Autodesk Inventor part; units mm, degrees
note: some values were not read from the file. Chosen so that the rebuilt part matches the saved one: direction of "Hole2".
(part 6 of 20)
  line L798 (-10086.965544, -10011.716706) -> (-10086.965599, -10011.716869)
  line L799 (-10086.460356, -10011.664008) -> (-10086.460302, -10011.663845)
  line L800 (-10067.443775, -10022.078908) -> (-10063.849959, -10021.096991)
  line L801 (-10063.849959, -10017.096991) -> (-10067.443775, -10016.115074)
  line L802 (-10063.849959, -10021.096991) -> (-10063.849959, -10017.096991)
  line L803 (-10064.171558, -10021.472431) -> (-10062.806719, -10021.096991)
  line L804 (-10062.806719, -10017.096991) -> (-10064.162196, -10016.724126)
  line L805 (-10062.806719, -10021.096991) -> (-10062.806719, -10017.096991)
  line L806 (-10064.538813, -10027.464433) -> (-10072.041452, -10028.601455)
  line L807 (-10064.538833, -10027.464382) -> (-10064.538813, -10027.464433)
  line L808 (-10072.041471, -10028.601404) -> (-10064.538833, -10027.464382)
  line L809 (-10072.041452, -10028.601455) -> (-10072.041471, -10028.601404)
  line L810 (-10064.074644, -10023.491407) -> (-10066.019072, -10022.707953)
  line L811 (-10064.074624, -10023.491459) -> (-10064.074644, -10023.491407)
  line L812 (-10077.559629, -10027.956681) -> (-10072.041471, -10028.601404)
  line L813 (-10077.559609, -10027.956732) -> (-10072.041452, -10028.601455)
  line L814 (-10064.538813, -10027.464433) -> (-10064.074624, -10023.491459)
  line L815 (-10064.538833, -10027.464382) -> (-10064.074644, -10023.491407)
  ellipse E634 centre (-10077.559589, -10027.956784) end of major axis (-10077.055021, -10028.015736) minor radius 0.000049 (-10077.55961, -10027.956732) -> (-10077.792591, -10027.929517) ccw
  ellipse E635 centre (-10077.559589, -10027.956784) end of major axis (-10076.550453, -10028.074688) minor radius 0.000097 (-10077.559631, -10027.956681) -> (-10078.025593, -10027.90225) ccw
  ellipse E636 centre (-10084.064431, -10027.197109) end of major axis (-10085.073566, -10027.079205) minor radius 0.000097 (-10084.530433, -10027.142576) -> (-10085.073566, -10027.079205) ccw
  ellipse E637 centre (-10084.064431, -10027.197109) end of major axis (-10084.568999, -10027.138157) minor radius 0.000049 (-10084.297432, -10027.169842) -> (-10084.568999, -10027.138157) ccw
  line L816 (-10085.073566, -10027.079205) -> (-10085.026899, -10026.679784)
  line L817 (-10077.79259, -10027.929517) -> (-10084.297432, -10027.169842)
  line L818 (-10078.025591, -10027.90225) -> (-10084.530433, -10027.142576)
  line L819 (-10085.073527, -10027.079306) -> (-10085.189452, -10028.072869)
  line L820 (-10084.684884, -10028.131821) -> (-10085.189452, -10028.072869)
  line L821 (-10084.684884, -10028.131821) -> (-10084.56896, -10027.138258)
  line L822 (-10085.073527, -10027.079306) -> (-10084.56896, -10027.138258)
  line L823 (-10085.189452, -10028.072869) -> (-10085.189425, -10028.072939)
  line L824 (-10084.56896, -10027.138258) -> (-10084.568999, -10027.138157)
  line L825 (-10085.073566, -10027.079205) -> (-10085.073527, -10027.079306)
  line L826 (-10065.745685, -10021.096991) -> (-10073.016339, -10023.096991)
  line L827 (-10065.804571, -10021.096991) -> (-10065.745685, -10021.096991)
  line L828 (-10073.075225, -10023.096991) -> (-10065.804571, -10021.096991)
  line L829 (-10073.016339, -10023.096991) -> (-10073.075225, -10023.096991)
  line L830 (-10073.016339, -10015.096991) -> (-10065.745685, -10017.096991)
  line L831 (-10073.075225, -10015.096991) -> (-10073.016339, -10015.096991)
  line L832 (-10065.804571, -10017.096991) -> (-10073.075225, -10015.096991)
  line L833 (-10065.745685, -10017.096991) -> (-10065.804571, -10017.096991)
  line L834 (-10078.593466, -10023.096991) -> (-10073.075225, -10023.096991)
  line L835 (-10078.593466, -10015.096991) -> (-10073.075225, -10015.096991)
  line L836 (-10065.745685, -10021.096991) -> (-10065.745685, -10017.096991)
  line L837 (-10065.804571, -10021.096991) -> (-10065.804571, -10017.096991)
  line L838 (-10078.593466, -10023.096991) -> (-10079.046133, -10023.096991)
  line L839 (-10078.593466, -10015.096991) -> (-10079.046133, -10015.096991)
  line L840 (-10079.046133, -10023.096991) -> (-10079.694033, -10023.096991)
  line L841 (-10079.694033, -10015.096991) -> (-10079.046133, -10015.096991)
  line L842 (-10085.400929, -10014.884409) -> (-10085.478798, -10015.096991)
  line L843 (-10084.974223, -10015.096991) -> (-10084.918326, -10014.944393)
  line L844 (-10085.478798, -10023.096991) -> (-10085.400929, -10023.309573)
  line L845 (-10084.918326, -10023.249589) -> (-10084.974223, -10023.096991)
  line L846 (-10064.074644, -10014.702574) -> (-10064.074624, -10014.702523)
  line L847 (-10066.019072, -10015.486029) -> (-10064.074644, -10014.702574)
  line L848 (-10072.041452, -10009.592527) -> (-10064.538813, -10010.729548)
  line L849 (-10072.041471, -10009.592578) -> (-10072.041452, -10009.592527)
  line L850 (-10064.538833, -10010.7296) -> (-10072.041471, -10009.592578)
  line L851 (-10064.538813, -10010.729548) -> (-10064.538833, -10010.7296)
  line L852 (-10072.041452, -10009.592527) -> (-10077.559609, -10010.237249)
  line L853 (-10077.559629, -10010.237301) -> (-10072.041471, -10009.592578)
  line L854 (-10064.074624, -10014.702523) -> (-10064.538813, -10010.729548)
  line L855 (-10064.074644, -10014.702574) -> (-10064.538833, -10010.7296)
  ellipse E638 centre (-10077.559589, -10010.237198) end of major axis (-10078.064157, -10010.29615) minor radius 0.000049 (-10077.79259, -10010.264465) -> (-10077.559609, -10010.237249) ccw
  ellipse E639 centre (-10077.559589, -10010.237198) end of major axis (-10076.550453, -10010.119294) minor radius 0.000097 (-10078.025593, -10010.291731) -> (-10077.559631, -10010.237301) ccw
  ellipse E640 centre (-10084.064431, -10010.996873) end of major axis (-10085.073566, -10011.114777) minor radius 0.000097 (-10085.073566, -10011.114777) -> (-10084.530433, -10011.051406) ccw
  ellipse E641 centre (-10084.064431, -10010.996873) end of major axis (-10084.568999, -10011.055825) minor radius 0.000049 (-10084.568999, -10011.055825) -> (-10084.297432, -10011.024139) ccw
  line L856 (-10085.026899, -10011.514198) -> (-10085.073566, -10011.114777)
  line L857 (-10077.79259, -10010.264465) -> (-10084.297432, -10011.024139)
  line L858 (-10084.530433, -10011.051406) -> (-10078.025591, -10010.291731)
  line L859 (-10085.189452, -10010.121112) -> (-10085.073527, -10011.114675)
  line L860 (-10084.56896, -10011.055724) -> (-10085.073527, -10011.114675)
  line L861 (-10084.56896, -10011.055724) -> (-10084.684884, -10010.06216)
  line L862 (-10084.684884, -10010.06216) -> (-10085.189452, -10010.121112)
  line L863 (-10085.189425, -10010.121042) -> (-10085.189452, -10010.121112)
  line L864 (-10085.073527, -10011.114675) -> (-10085.073566, -10011.114777)
  line L865 (-10084.568999, -10011.055825) -> (-10084.56896, -10011.055724)
  line L866 (-10081.349998, -10026.695676) -> (-10079.440529, -10026.876667)
  line L867 (-10081.349996, -10026.695712) -> (-10080.62193, -10026.764723)
  ellipse E642 centre (-10081.349994, -10026.695749) end of major axis (-10080.84426, -10026.743685) minor radius 0.000036 (-10081.349998, -10026.695712) -> (-10081.583519, -10026.673581) ccw
  ellipse E643 centre (-10081.349994, -10026.695749) end of major axis (-10080.338527, -10026.791622) minor radius 0.000072 (-10081.350003, -10026.695675) -> (-10081.817045, -10026.651414) ccw
  ellipse E644 centre (-10087.869978, -10026.077987) end of major axis (-10088.881445, -10025.982114) minor radius 0.000072 (-10088.337025, -10026.033654) -> (-10088.881445, -10025.982114) ccw
  ellipse E645 centre (-10087.869978, -10026.077987) end of major axis (-10088.375711, -10026.030051) minor radius 0.000036 (-10088.103502, -10026.05582) -> (-10088.375711, -10026.030051) ccw
  line L868 (-10088.881445, -10025.982114) -> (-10088.665315, -10023.701932)
  line L869 (-10081.583517, -10026.673582) -> (-10088.103502, -10026.05582)
  line L870 (-10081.817041, -10026.651415) -> (-10088.337025, -10026.033654)
  line L871 (-10088.88144, -10025.982186) -> (-10088.975789, -10026.97795)
  line L872 (-10088.470056, -10027.025887) -> (-10088.975789, -10026.97795)
  line L873 (-10088.470056, -10027.025887) -> (-10088.375707, -10026.030122)
  line L874 (-10088.88144, -10025.982186) -> (-10088.375707, -10026.030122)
  line L875 (-10088.975789, -10026.97795) -> (-10088.975783, -10026.978063)
  line L876 (-10088.375707, -10026.030122) -> (-10088.375711, -10026.030051)
  line L877 (-10088.881445, -10025.982114) -> (-10088.88144, -10025.982186)
  line L878 (-10082.191609, -10023.096991) -> (-10081.297088, -10023.096991)
  line L879 (-10082.191609, -10015.096991) -> (-10081.297088, -10015.096991)
  line L880 (-10082.191609, -10023.096991) -> (-10082.647825, -10023.096991)
  line L881 (-10082.191609, -10015.096991) -> (-10082.647825, -10015.096991)
  line L882 (-10088.846266, -10015.096991) -> (-10089.310215, -10015.096991)
  line L883 (-10089.310215, -10023.096991) -> (-10088.846266, -10023.096991)
  line L884 (-10089.310215, -10023.096991) -> (-10089.310215, -10015.096991)
  line L885 (-10082.647825, -10023.096991) -> (-10088.846266, -10023.096991)
  line L886 (-10088.846266, -10015.096991) -> (-10082.647825, -10015.096991)
  line L887 (-10088.913293, -10014.096991) -> (-10089.21136, -10015.096991)
  line L888 (-10088.705625, -10015.096991) -> (-10088.563509, -10014.620199)
  line L889 (-10088.702761, -10014.096991) -> (-10088.913293, -10014.096991)
  line L890 (-10089.21136, -10023.096991) -> (-10088.913293, -10024.096991)
  line L891 (-10088.702761, -10024.096991) -> (-10088.913293, -10024.096991)
  line L892 (-10088.563509, -10023.573783) -> (-10088.705625, -10023.096991)
  line L893 (-10080.62193, -10011.429259) -> (-10081.349996, -10011.498269)
  line L894 (-10081.349998, -10011.498306) -> (-10079.440529, -10011.317315)
  ellipse E646 centre (-10081.349994, -10011.498233) end of major axis (-10081.855727, -10011.54617) minor radius 0.000036 (-10081.583517, -10011.5204) -> (-10081.349996, -10011.498269) ccw
  ellipse E647 centre (-10081.349994, -10011.498233) end of major axis (-10080.338527, -10011.40236) minor radius 0.000072 (-10081.817045, -10011.542567) -> (-10081.350003, -10011.498306) ccw
  ellipse E648 centre (-10087.869978, -10012.115994) end of major axis (-10088.881445, -10012.211867) minor radius 0.000072 (-10088.881445, -10012.211867) -> (-10088.337025, -10012.160328) ccw
  ellipse E649 centre (-10087.869978, -10012.115994) end of major axis (-10088.375711, -10012.163931) minor radius 0.000036 (-10088.375711, -10012.163931) -> (-10088.103502, -10012.138161) ccw
  line L895 (-10088.665315, -10014.492049) -> (-10088.881445, -10012.211867)
  line L896 (-10081.583517, -10011.5204) -> (-10088.103502, -10012.138161)
  line L897 (-10088.337025, -10012.160328) -> (-10081.817041, -10011.542567)
  line L898 (-10088.975789, -10011.216032) -> (-10088.88144, -10012.211796)
  line L899 (-10088.375707, -10012.163859) -> (-10088.88144, -10012.211796)
  line L900 (-10088.375707, -10012.163859) -> (-10088.470056, -10011.168095)
  line L901 (-10088.470056, -10011.168095) -> (-10088.975789, -10011.216032)
  line L902 (-10088.975783, -10011.215919) -> (-10088.975789, -10011.216032)
  line L903 (-10088.88144, -10012.211796) -> (-10088.881445, -10012.211867)
  line L904 (-10088.375711, -10012.163931) -> (-10088.375707, -10012.163859)
  line L905 (-10077.691531, -10026.87864) -> (-10077.890346, -10026.857838)
  line L906 (-10077.890422, -10026.85761) -> (-10077.691508, -10026.878422)
  line L907 (-10077.890346, -10026.857838) -> (-10077.890422, -10026.85761)
  line L908 (-10077.717522, -10027.127065) -> (-10077.717446, -10027.127293)
  line L909 (-10077.691508, -10026.878422) -> (-10077.717522, -10027.127065)
  line L910 (-10077.58745, -10025.883851) -> (-10077.786364, -10025.863039)
  line L911 (-10077.561436, -10025.635208) -> (-10077.58745, -10025.883851)
  line L912 (-10075.671674, -10025.833146) -> (-10075.697666, -10026.081571)
  line L913 (-10075.67175, -10025.832918) -> (-10075.671674, -10025.833146)
  line L914 (-10075.49885, -10026.102372) -> (-10075.697765, -10026.081561)
  line L915 (-10075.697765, -10026.081561) -> (-10075.67175, -10025.832918)
  line L916 (-10075.498774, -10026.1026) -> (-10075.49885, -10026.102372)
  line L917 (-10075.498774, -10026.1026) -> (-10075.526412, -10026.366754)
  line L918 (-10075.973217, -10027.309784) -> (-10077.717446, -10027.127293)
  line L919 (-10077.890422, -10026.85761) -> (-10077.786364, -10025.863039)
  line L920 (-10077.561436, -10025.635208) -> (-10075.67175, -10025.832918)
  line L921 (-10075.827837, -10027.324775) -> (-10077.717522, -10027.127065)
  line L922 (-10075.49885, -10026.102372) -> (-10075.602908, -10027.096943)
  line L923 (-10075.827837, -10027.324775) -> (-10075.801822, -10027.076132)
  line L924 (-10075.801822, -10027.076132) -> (-10075.602908, -10027.096943)
  line L925 (-10077.388536, -10025.904662) -> (-10075.896679, -10026.060749)
  line L926 (-10075.896679, -10026.060749) -> (-10076.000737, -10027.05532)
  line L927 (-10076.000737, -10027.05532) -> (-10077.492594, -10026.899234)
  line L928 (-10077.492594, -10026.899234) -> (-10077.388536, -10025.904662)
  line L929 (-10076.090343, -10026.217933) -> (-10077.23146, -10026.098543)
  line L930 (-10075.896679, -10026.060749) -> (-10076.090343, -10026.217933)
  line L931 (-10077.388536, -10025.904662) -> (-10077.23146, -10026.098543)
  line L932 (-10077.23146, -10026.098543) -> (-10077.298821, -10026.742375)
  line L933 (-10077.492594, -10026.899234) -> (-10077.298821, -10026.742375)
  line L934 (-10077.298821, -10026.742375) -> (-10076.157704, -10026.861765)
  line L935 (-10076.000737, -10027.05532) -> (-10076.157704, -10026.861765)
  line L936 (-10076.157704, -10026.861765) -> (-10076.090343, -10026.217933)
  circle A21 centre (-10076.955085, -10026.45286) radius 0.1
  line L937 (-10076.809659, -10026.618901) -> (-10077.131723, -10026.585205)
  line L938 (-10077.131713, -10026.585238) -> (-10077.131723, -10026.585205)
  line L939 (-10076.809648, -10026.618934) -> (-10077.131713, -10026.585238)
  line L940 (-10076.809648, -10026.618934) -> (-10076.809659, -10026.618901)
  line L941 (-10077.131723, -10026.585205) -> (-10077.100506, -10026.286834)
  line L942 (-10077.100506, -10026.286834) -> (-10076.778441, -10026.32053)
  line L943 (-10076.77843, -10026.320563) -> (-10076.778441, -10026.32053)
  line L944 (-10076.778441, -10026.32053) -> (-10076.809659, -10026.618901)
  line L945 (-10076.77843, -10026.320563) -> (-10076.809648, -10026.618934)
  line L946 (-10067.064443, -10025.491943) -> (-10067.085254, -10025.690857)
  line L947 (-10067.064519, -10025.491715) -> (-10067.064443, -10025.491943)
  line L948 (-10067.08533, -10025.690629) -> (-10067.064519, -10025.491715)
  line L949 (-10067.085254, -10025.690857) -> (-10067.08533, -10025.690629)
  line L950 (-10066.8158, -10025.517958) -> (-10067.064443, -10025.491943)
  line L951 (-10066.815876, -10025.51773) -> (-10066.8158, -10025.517958)
  line L952 (-10067.064519, -10025.491715) -> (-10066.815876, -10025.51773)
  line L953 (-10068.059113, -10025.387875) -> (-10068.307657, -10025.361871)
  line L954 (-10068.079902, -10025.586572) -> (-10068.079826, -10025.5868)
  line L955 (-10068.05909, -10025.387657) -> (-10068.079902, -10025.586572)
  line L956 (-10068.307733, -10025.361643) -> (-10068.05909, -10025.387657)
  line L957 (-10068.307657, -10025.361871) -> (-10068.307733, -10025.361643)
  line L958 (-10067.085254, -10025.690857) -> (-10068.079826, -10025.5868)
  line L959 (-10066.61809, -10023.628272) -> (-10066.8158, -10025.517958)
  line L960 (-10067.08533, -10025.690629) -> (-10068.079902, -10025.586572)
  line L961 (-10068.307733, -10025.361643) -> (-10068.110023, -10023.471958)
  line L962 (-10066.618166, -10023.628044) -> (-10066.815876, -10025.51773)
  line L963 (-10067.840569, -10023.299058) -> (-10066.845997, -10023.403116)
  line L964 (-10066.845921, -10023.403344) -> (-10066.86671, -10023.60204)
  line L965 (-10066.618166, -10023.628044) -> (-10066.866809, -10023.60203)
  line L966 (-10066.866809, -10023.60203) -> (-10066.845997, -10023.403116)
  line L967 (-10066.845997, -10023.403116) -> (-10066.845921, -10023.403344)
  line L968 (-10066.61809, -10023.628272) -> (-10066.618166, -10023.628044)
  line L969 (-10067.840569, -10023.299058) -> (-10067.86138, -10023.497972)
  line L970 (-10067.86138, -10023.497972) -> (-10068.110023, -10023.471958)
  line L971 (-10068.038279, -10025.188743) -> (-10067.882192, -10023.696886)
  line L972 (-10067.882192, -10023.696886) -> (-10066.887621, -10023.800944)
  line L973 (-10066.887621, -10023.800944) -> (-10067.043707, -10025.292801)
  line L974 (-10067.043707, -10025.292801) -> (-10068.038279, -10025.188743)
  line L975 (-10067.725116, -10023.890767) -> (-10067.844506, -10025.031884)
  line L976 (-10067.882192, -10023.696886) -> (-10067.725116, -10023.890767)
  line L977 (-10068.038279, -10025.188743) -> (-10067.844506, -10025.031884)
  line L978 (-10067.844506, -10025.031884) -> (-10067.200675, -10025.099246)
  line L979 (-10067.043707, -10025.292801) -> (-10067.200675, -10025.099246)
  line L980 (-10067.200675, -10025.099246) -> (-10067.081284, -10023.958128)
  line L981 (-10066.887621, -10023.800944) -> (-10067.081284, -10023.958128)
  line L982 (-10067.081284, -10023.958128) -> (-10067.725116, -10023.890767)
  circle A22 centre (-10067.490163, -10024.755455) radius 0.1
  line L983 (-10067.324126, -10024.61004) -> (-10067.357823, -10024.932104)
  line L984 (-10067.357812, -10024.932137) -> (-10067.357823, -10024.932104)
  line L985 (-10067.324115, -10024.610072) -> (-10067.357812, -10024.932137)
  line L986 (-10067.324115, -10024.610072) -> (-10067.324126, -10024.61004)
  line L987 (-10067.357823, -10024.932104) -> (-10067.656194, -10024.900887)
  line L988 (-10067.656183, -10024.90092) -> (-10067.656194, -10024.900887)
  line L989 (-10067.357812, -10024.932137) -> (-10067.656183, -10024.90092)
  line L990 (-10067.656194, -10024.900887) -> (-10067.622498, -10024.578822)
  line L991 (-10067.622498, -10024.578822) -> (-10067.324126, -10024.61004)
  line L992 (-10079.023383, -10022.531991) -> (-10078.824469, -10022.531991)
  line L993 (-10078.824469, -10022.531991) -> (-10078.824469, -10022.781991)
  line L994 (-10078.824469, -10021.531991) -> (-10079.023383, -10021.531991)
  line L995 (-10078.824469, -10021.281991) -> (-10078.824469, -10021.531991)
  line L996 (-10079.023383, -10022.531991) -> (-10079.023383, -10021.531991)
  line L997 (-10078.824469, -10021.281991) -> (-10077.066524, -10021.281991)
  line L998 (-10077.066524, -10022.781991) -> (-10078.824469, -10022.781991)
  line L999 (-10078.625555, -10021.531991) -> (-10077.265175, -10021.531991)
  line L1000 (-10077.265175, -10022.531991) -> (-10078.625555, -10022.531991)
  line L1001 (-10078.625555, -10022.531991) -> (-10078.625555, -10021.531991)
  line L1002 (-10078.625555, -10021.531991) -> (-10078.372051, -10021.691952)
  line L1003 (-10078.625555, -10022.531991) -> (-10078.372051, -10022.37203)
  ellipse E650 centre (-10078.062063, -10022.031991) end of major axis (-10078.062063, -10021.931991) minor radius 0.099457
  ellipse E651 centre (-10078.056859, -10022.031991) end of major axis (-10078.056859, -10021.931991) minor radius 0.099457 (-10078.056859, -10022.131991) -> (-10078.056859, -10021.931991) ccw
  line L1004 (-10078.056859, -10022.131991) -> (-10078.062063, -10022.131991)
  line L1005 (-10078.056859, -10021.931991) -> (-10078.062063, -10021.931991)
  line L1006 (-10077.895827, -10022.181991) -> (-10078.217892, -10022.181991)
  line L1007 (-10077.88528, -10022.181991) -> (-10077.895827, -10022.181991)
  line L1008 (-10078.217892, -10022.181991) -> (-10078.217892, -10021.881991)
  line L1009 (-10078.217892, -10021.881991) -> (-10077.895827, -10021.881991)
  line L1010 (-10077.88528, -10021.881991) -> (-10077.895827, -10021.881991)
  line L1011 (-10077.895827, -10021.881991) -> (-10077.895827, -10022.181991)
  line L1012 (-10068.456079, -10020.246991) -> (-10068.456079, -10020.046991)
  line L1013 (-10068.374152, -10020.246991) -> (-10068.456079, -10020.246991)
  line L1014 (-10068.207437, -10020.046991) -> (-10068.12582, -10020.046991)
  line L1015 (-10068.456079, -10020.046991) -> (-10068.207437, -10020.046991)
  line L1016 (-10069.450649, -10020.046991) -> (-10069.450649, -10020.246991)
  line L1017 (-10069.699291, -10020.046991) -> (-10069.450649, -10020.046991)
  line L1018 (-10068.456079, -10020.246991) -> (-10069.450649, -10020.246991)
  line L1019 (-10069.699291, -10020.046991) -> (-10069.699291, -10018.146991)
  line L1020 (-10068.207437, -10018.146991) -> (-10068.207437, -10020.046991)
  line L1021 (-10069.450649, -10017.946991) -> (-10068.456079, -10017.946991)
  line L1022 (-10068.207437, -10018.146991) -> (-10068.456079, -10018.146991)
  line L1023 (-10068.456079, -10018.146991) -> (-10068.456079, -10017.946991)
  line L1024 (-10068.456079, -10017.946991) -> (-10068.374152, -10017.946991)
  line L1025 (-10068.12582, -10018.146991) -> (-10068.207437, -10018.146991)
  line L1026 (-10069.450649, -10017.946991) -> (-10069.450649, -10018.146991)
  line L1027 (-10069.450649, -10018.146991) -> (-10069.699291, -10018.146991)
  line L1028 (-10069.450649, -10019.846991) -> (-10069.450649, -10018.346991)
  line L1029 (-10069.450649, -10018.346991) -> (-10068.456079, -10018.346991)
  line L1030 (-10068.456079, -10018.346991) -> (-10068.456079, -10019.846991)
  line L1031 (-10068.456079, -10019.846991) -> (-10069.450649, -10019.846991)
  line L1032 (-10069.450649, -10018.346991) -> (-10069.227806, -10018.487604)
  line L1033 (-10069.450649, -10019.846991) -> (-10069.227806, -10019.706378)
  line L1034 (-10068.456079, -10019.846991) -> (-10068.512324, -10019.707891)
  line L1035 (-10068.456079, -10018.346991) -> (-10068.512324, -10018.48609)
  ellipse E652 centre (-10068.87531, -10019.358902) end of major axis (-10068.87531, -10019.258902) minor radius 0.099457
  line L1036 (-10068.870817, -10019.458902) -> (-10068.87531, -10019.458902)
  line L1037 (-10068.870817, -10019.258902) -> (-10068.87531, -10019.258902)
  line L1038 (-10066.86671, -10014.591942) -> (-10066.845921, -10014.790638)
  line L1039 (-10066.845997, -10014.790866) -> (-10066.866809, -10014.591952)
  line L1040 (-10066.845921, -10014.790638) -> (-10066.845997, -10014.790866)
  line L1041 (-10066.618166, -10014.565937) -> (-10066.61809, -10014.565709)
  line L1042 (-10066.866809, -10014.591952) -> (-10066.618166, -10014.565937)
  line L1043 (-10067.86138, -10014.69601) -> (-10067.840569, -10014.894924)
  line L1044 (-10068.110023, -10014.722024) -> (-10067.86138, -10014.69601)
  line L1045 (-10068.307657, -10012.832111) -> (-10068.059113, -10012.806107)
  line L1046 (-10068.307733, -10012.832339) -> (-10068.307657, -10012.832111)
  line L1047 (-10068.079902, -10012.60741) -> (-10068.05909, -10012.806324)
  line L1048 (-10068.05909, -10012.806324) -> (-10068.307733, -10012.832339)
  line L1049 (-10068.079826, -10012.607182) -> (-10068.079902, -10012.60741)
  line L1050 (-10068.079826, -10012.607182) -> (-10067.085254, -10012.503124)
  line L1051 (-10066.8158, -10012.676024) -> (-10066.61809, -10014.565709)
  line L1052 (-10066.845997, -10014.790866) -> (-10067.840569, -10014.894924)
  line L1053 (-10068.110023, -10014.722024) -> (-10068.307733, -10012.832339)
  line L1054 (-10066.815876, -10012.676252) -> (-10066.618166, -10014.565937)
  line L1055 (-10068.079902, -10012.60741) -> (-10067.08533, -10012.503352)
  line L1056 (-10067.085254, -10012.503124) -> (-10067.064443, -10012.702038)
  line L1057 (-10067.064443, -10012.702038) -> (-10066.8158, -10012.676024)
  line L1058 (-10066.815876, -10012.676252) -> (-10067.064519, -10012.702267)
  line L1059 (-10067.064519, -10012.702267) -> (-10067.08533, -10012.503352)
  line L1060 (-10067.08533, -10012.503352) -> (-10067.085254, -10012.503124)
  line L1061 (-10067.064519, -10012.702267) -> (-10067.064443, -10012.702038)
  line L1062 (-10066.8158, -10012.676024) -> (-10066.815876, -10012.676252)
  line L1063 (-10067.882192, -10014.497095) -> (-10068.038279, -10013.005239)
  line L1064 (-10068.038279, -10013.005239) -> (-10067.043707, -10012.901181)
  line L1065 (-10067.043707, -10012.901181) -> (-10066.887621, -10014.393038)
  line L1066 (-10066.887621, -10014.393038) -> (-10067.882192, -10014.497095)
  line L1067 (-10067.844506, -10013.162097) -> (-10067.725116, -10014.303215)
  line L1068 (-10068.038279, -10013.005239) -> (-10067.844506, -10013.162097)
  line L1069 (-10067.882192, -10014.497095) -> (-10067.725116, -10014.303215)
  line L1070 (-10067.725116, -10014.303215) -> (-10067.081284, -10014.235853)
  line L1071 (-10066.887621, -10014.393038) -> (-10067.081284, -10014.235853)
  line L1072 (-10067.081284, -10014.235853) -> (-10067.200675, -10013.094736)
  line L1073 (-10067.043707, -10012.901181) -> (-10067.200675, -10013.094736)
  line L1074 (-10067.200675, -10013.094736) -> (-10067.844506, -10013.162097)
  circle A23 centre (-10067.435655, -10013.959505) radius 0.1
  line L1075 (-10067.303315, -10013.782856) -> (-10067.269618, -10014.104921)
  line L1076 (-10067.269608, -10014.104888) -> (-10067.269618, -10014.104921)
  line L1077 (-10067.303304, -10013.782824) -> (-10067.269608, -10014.104888)
  line L1078 (-10067.303304, -10013.782824) -> (-10067.303315, -10013.782856)
  line L1079 (-10067.269618, -10014.104921) -> (-10067.56799, -10014.136138)
  line L1080 (-10067.56799, -10014.136138) -> (-10067.601686, -10013.814074)
  line L1081 (-10067.601675, -10013.814041) -> (-10067.601686, -10013.814074)
  line L1082 (-10067.601686, -10013.814074) -> (-10067.303315, -10013.782856)
  line L1083 (-10067.601675, -10013.814041) -> (-10067.303304, -10013.782824)
  line L1084 (-10064.599959, -10020.246991) -> (-10064.599959, -10020.046991)
  line L1085 (-10064.599959, -10020.046991) -> (-10064.349959, -10020.046991)
  line L1086 (-10065.599959, -10020.046991) -> (-10065.599959, -10020.246991)
  line L1087 (-10065.745685, -10020.046991) -> (-10065.599959, -10020.046991)
  line L1088 (-10064.599959, -10020.246991) -> (-10065.599959, -10020.246991)
  line L1089 (-10064.349959, -10018.146991) -> (-10064.349959, -10020.046991)
  line L1090 (-10065.599959, -10017.946991) -> (-10064.599959, -10017.946991)
  line L1091 (-10064.349959, -10018.146991) -> (-10064.599959, -10018.146991)
  line L1092 (-10064.599959, -10018.146991) -> (-10064.599959, -10017.946991)
  line L1093 (-10065.599959, -10017.946991) -> (-10065.599959, -10018.146991)
  line L1094 (-10065.599959, -10018.146991) -> (-10065.745685, -10018.146991)
  line L1095 (-10065.599959, -10019.846991) -> (-10065.599959, -10018.346991)
  line L1096 (-10065.599959, -10018.346991) -> (-10064.599959, -10018.346991)
  line L1097 (-10064.599959, -10018.346991) -> (-10064.599959, -10019.846991)
  line L1098 (-10064.599959, -10019.846991) -> (-10065.599959, -10019.846991)
  line L1099 (-10065.423632, -10018.523318) -> (-10065.423632, -10019.670664)
  line L1100 (-10065.599959, -10018.346991) -> (-10065.423632, -10018.523318)
  line L1101 (-10065.599959, -10019.846991) -> (-10065.423632, -10019.670664)
  line L1102 (-10065.423632, -10019.670664) -> (-10064.776286, -10019.670664)
  line L1103 (-10064.599959, -10019.846991) -> (-10064.776286, -10019.670664)
  line L1104 (-10064.776286, -10019.670664) -> (-10064.776286, -10018.523318)
  line L1105 (-10064.599959, -10018.346991) -> (-10064.776286, -10018.523318)
  line L1106 (-10064.776286, -10018.523318) -> (-10065.423632, -10018.523318)
  circle A24 centre (-10065.099959, -10019.358902) radius 0.1
  line L1107 (-10064.949959, -10019.196991) -> (-10064.949959, -10019.520814)
  line L1108 (-10064.949959, -10019.520814) -> (-10065.249959, -10019.520814)
  line L1109 (-10065.249959, -10019.520814) -> (-10065.249959, -10019.196991)
  line L1110 (-10065.249959, -10019.196991) -> (-10064.949959, -10019.196991)
  line L1111 (-10063.389287, -10020.246991) -> (-10063.389287, -10020.046991)
  line L1112 (-10063.389287, -10020.046991) -> (-10063.140974, -10020.046991)
  line L1113 (-10063.389287, -10020.246991) -> (-10063.849959, -10020.246991)
  line L1114 (-10063.140974, -10018.146991) -> (-10063.140974, -10020.046991)
  line L1115 (-10063.849959, -10017.946991) -> (-10063.389287, -10017.946991)
  line L1116 (-10063.140974, -10018.146991) -> (-10063.389287, -10018.146991)
  line L1117 (-10063.389287, -10018.146991) -> (-10063.389287, -10017.946991)
  line L1118 (-10063.849959, -10018.346991) -> (-10063.389287, -10018.346991)
  line L1119 (-10063.389287, -10018.346991) -> (-10063.389287, -10019.846991)
  line L1120 (-10063.389287, -10019.846991) -> (-10063.849959, -10019.846991)
  line L1121 (-10063.849959, -10019.670664) -> (-10063.680403, -10019.670664)
  line L1122 (-10063.389287, -10019.846991) -> (-10063.680403, -10019.670664)
  line L1123 (-10063.680403, -10019.670664) -> (-10063.680403, -10018.523318)
  line L1124 (-10063.389287, -10018.346991) -> (-10063.680403, -10018.523318)
  line L1125 (-10063.680403, -10018.523318) -> (-10063.849959, -10018.523318)
  line L1126 (-10063.829708, -10019.196991) -> (-10063.829708, -10019.520814)
  line L1127 (-10063.829708, -10019.520814) -> (-10063.849959, -10019.520814)
  line L1128 (-10063.849959, -10019.196991) -> (-10063.829708, -10019.196991)
  line L1129 (-10076.003562, -10027.569508) -> (-10075.804914, -10027.592717)
  line L1130 (-10076.003508, -10027.569649) -> (-10076.003562, -10027.569508)
  line L1131 (-10075.833925, -10027.841028) -> (-10075.833871, -10027.84117)
  line L1132 (-10075.804914, -10027.592717) -> (-10075.833925, -10027.841028)
  line L1133 (-10073.715814, -10027.808888) -> (-10073.719047, -10027.836558)
  line L1134 (-10073.946708, -10028.06166) -> (-10075.833871, -10027.84117)
  line L1135 (-10076.003562, -10027.569508) -> (-10075.973192, -10027.309567)
  line L1136 (-10075.52651, -10026.366742) -> (-10073.772692, -10026.571653)
  line L1137 (-10073.946762, -10028.061518) -> (-10075.833925, -10027.841028)
  line L1138 (-10073.603055, -10026.843173) -> (-10073.719102, -10027.836417)
  line L1139 (-10073.719047, -10027.836558) -> (-10073.815719, -10027.825263)
  line L1140 (-10073.920953, -10027.841223) -> (-10073.946708, -10028.06166)
  line L1141 (-10073.946762, -10028.061518) -> (-10073.917751, -10027.813207)
  line L1142 (-10073.917751, -10027.813207) -> (-10073.719102, -10027.836417)
  line L1143 (-10073.719102, -10027.836417) -> (-10073.719047, -10027.836558)
  line L1144 (-10073.917751, -10027.813207) -> (-10073.917696, -10027.813348)
  line L1145 (-10073.946708, -10028.06166) -> (-10073.946762, -10028.061518)
  line L1146 (-10073.772692, -10026.571653) -> (-10073.772637, -10026.571794)
  line L1147 (-10073.603055, -10026.843173) -> (-10073.801703, -10026.819963)
  line L1148 (-10073.801703, -10026.819963) -> (-10073.772692, -10026.571653)
  line L1149 (-10073.603, -10026.843314) -> (-10073.603055, -10026.843173)
  line L1150 (-10075.490218, -10026.622683) -> (-10074.000352, -10026.796754)
  line L1151 (-10074.000352, -10026.796754) -> (-10074.116399, -10027.789998)
  line L1152 (-10074.116399, -10027.789998) -> (-10075.606265, -10027.615927)
  line L1153 (-10075.606265, -10027.615927) -> (-10075.490218, -10026.622683)
  line L1154 (-10074.195911, -10026.951529) -> (-10075.335505, -10026.818382)
  line L1155 (-10074.000352, -10026.796754) -> (-10074.195911, -10026.951529)
  line L1156 (-10075.490218, -10026.622683) -> (-10075.335505, -10026.818382)
  line L1157 (-10075.335505, -10026.818382) -> (-10075.410628, -10027.461355)
  line L1158 (-10075.606265, -10027.615927) -> (-10075.410628, -10027.461355)
  line L1159 (-10075.410628, -10027.461355) -> (-10074.271034, -10027.594501)
  line L1160 (-10074.116399, -10027.789998) -> (-10074.271034, -10027.594501)
  line L1161 (-10074.271034, -10027.594501) -> (-10074.195911, -10026.951529)
  circle A25 centre (-10075.063421, -10027.176022) radius 0.1
  line L1162 (-10074.920009, -10027.343803) -> (-10075.241644, -10027.306224)
  line L1163 (-10075.241636, -10027.306245) -> (-10075.241644, -10027.306224)
  line L1164 (-10074.920001, -10027.343823) -> (-10075.241636, -10027.306245)
  line L1165 (-10074.920001, -10027.343823) -> (-10074.920009, -10027.343803)
  line L1166 (-10075.241644, -10027.306224) -> (-10075.20683, -10027.008251)
  line L1167 (-10075.20683, -10027.008251) -> (-10074.885195, -10027.04583)
  line L1168 (-10074.885187, -10027.04585) -> (-10074.885195, -10027.04583)
  line L1169 (-10074.885195, -10027.04583) -> (-10074.920009, -10027.343803)
  line L1170 (-10074.885187, -10027.04585) -> (-10074.920001, -10027.343823)
  line L1171 (-10065.161916, -10026.334441) -> (-10065.185126, -10026.53309)
  line L1172 (-10065.161971, -10026.334299) -> (-10065.161916, -10026.334441)
  line L1173 (-10065.18518, -10026.532948) -> (-10065.161971, -10026.334299)
  line L1174 (-10065.185126, -10026.53309) -> (-10065.18518, -10026.532948)
  line L1175 (-10064.913605, -10026.363453) -> (-10065.161916, -10026.334441)
  line L1176 (-10064.91366, -10026.363311) -> (-10064.913605, -10026.363453)
  line L1177 (-10065.161971, -10026.334299) -> (-10064.91366, -10026.363311)
  line L1178 (-10066.15523, -10026.218385) -> (-10066.383563, -10026.191708)
  line L1179 (-10066.178424, -10026.416901) -> (-10066.178369, -10026.417042)
  line L1180 (-10066.155214, -10026.218252) -> (-10066.178424, -10026.416901)
  line L1181 (-10066.403525, -10026.18924) -> (-10066.155214, -10026.218252)
  line L1182 (-10066.403471, -10026.189382) -> (-10066.403525, -10026.18924)
  line L1183 (-10065.185126, -10026.53309) -> (-10066.178369, -10026.417042)
  line L1184 (-10064.693115, -10024.47629) -> (-10064.913605, -10026.363453)
  line L1185 (-10065.18518, -10026.532948) -> (-10066.178424, -10026.416901)
  line L1186 (-10066.403525, -10026.18924) -> (-10066.183036, -10024.302077)
  line L1187 (-10064.69317, -10024.476148) -> (-10064.91366, -10026.363311)
  line L1188 (-10065.911515, -10024.13244) -> (-10064.918271, -10024.248488)
  line L1189 (-10064.918217, -10024.248629) -> (-10064.941411, -10024.447144)
  line L1190 (-10064.69317, -10024.476148) -> (-10064.941481, -10024.447136)
  line L1191 (-10064.941481, -10024.447136) -> (-10064.918271, -10024.248488)
  line L1192 (-10064.918271, -10024.248488) -> (-10064.918217, -10024.248629)
  line L1193 (-10064.693115, -10024.47629) -> (-10064.69317, -10024.476148)
  line L1194 (-10065.911515, -10024.13244) -> (-10065.934725, -10024.331089)
  line L1195 (-10065.934725, -10024.331089) -> (-10066.183036, -10024.302077)
  line L1196 (-10066.132005, -10026.019603) -> (-10065.957934, -10024.529738)
  line L1197 (-10065.957934, -10024.529738) -> (-10064.96469, -10024.645785)
  line L1198 (-10064.96469, -10024.645785) -> (-10065.138761, -10026.135651)
  line L1199 (-10065.138761, -10026.135651) -> (-10066.132005, -10026.019603)
  line L1200 (-10065.803222, -10024.725437) -> (-10065.936368, -10025.865031)
  line L1201 (-10065.957934, -10024.529738) -> (-10065.803222, -10024.725437)
  line L1202 (-10066.132005, -10026.019603) -> (-10065.936368, -10025.865031)
  line L1203 (-10065.936368, -10025.865031) -> (-10065.293396, -10025.940154)
  line L1204 (-10065.138761, -10026.135651) -> (-10065.293396, -10025.940154)
  line L1205 (-10065.293396, -10025.940154) -> (-10065.160249, -10024.80056)
  line L1206 (-10064.96469, -10024.645785) -> (-10065.160249, -10024.80056)
  line L1207 (-10065.160249, -10024.80056) -> (-10065.803222, -10024.725437)
  circle A26 centre (-10065.578713, -10025.592912) radius 0.1
  line L1208 (-10065.410935, -10025.449506) -> (-10065.448513, -10025.771141)
  line L1209 (-10065.448506, -10025.771162) -> (-10065.448513, -10025.771141)
  line L1210 (-10065.410927, -10025.449527) -> (-10065.448506, -10025.771162)
  line L1211 (-10065.410927, -10025.449527) -> (-10065.410935, -10025.449506)
  line L1212 (-10065.448513, -10025.771141) -> (-10065.746487, -10025.736327)
  line L1213 (-10065.746479, -10025.736347) -> (-10065.746487, -10025.736327)
  line L1214 (-10065.448506, -10025.771162) -> (-10065.746479, -10025.736347)
  line L1215 (-10065.746487, -10025.736327) -> (-10065.708908, -10025.414692)
  line L1216 (-10065.708908, -10025.414692) -> (-10065.410935, -10025.449506)
  line L1217 (-10077.265175, -10022.531991) -> (-10077.066524, -10022.531991)
  line L1218 (-10077.066524, -10022.531991) -> (-10077.066524, -10022.781991)
  line L1219 (-10077.066524, -10021.531991) -> (-10077.265175, -10021.531991)
  line L1220 (-10077.066524, -10021.281991) -> (-10077.066524, -10021.531991)
  line L1221 (-10075.017046, -10021.281991) -> (-10075.017046, -10021.531991)
  line L1222 (-10075.179332, -10021.281991) -> (-10075.017046, -10021.281991)
  line L1223 (-10074.98068, -10021.531991) -> (-10075.179332, -10021.531991)
  line L1224 (-10075.179332, -10021.531991) -> (-10075.179332, -10021.281991)
  line L1225 (-10074.818395, -10021.531991) -> (-10074.98068, -10021.531991)
  line L1226 (-10074.818395, -10021.531991) -> (-10074.818395, -10022.531991)
  line L1227 (-10077.265175, -10022.531991) -> (-10077.265175, -10021.531991)
  line L1228 (-10077.066524, -10021.281991) -> (-10075.179332, -10021.281991)
  line L1229 (-10075.179332, -10022.781991) -> (-10077.066524, -10022.781991)
  line L1230 (-10074.98068, -10021.531991) -> (-10074.98068, -10022.531991)
  line L1231 (-10075.017046, -10022.531991) -> (-10075.017046, -10022.781991)
  line L1232 (-10075.179332, -10022.781991) -> (-10075.179332, -10022.531991)
  line L1233 (-10075.179332, -10022.531991) -> (-10074.98068, -10022.531991)
  line L1234 (-10074.98068, -10022.531991) -> (-10074.818395, -10022.531991)
  line L1235 (-10075.017046, -10022.781991) -> (-10075.179332, -10022.781991)
  line L1236 (-10076.867872, -10021.531991) -> (-10075.377984, -10021.531991)
  line L1237 (-10075.377984, -10021.531991) -> (-10075.377984, -10022.531991)
  line L1238 (-10075.377984, -10022.531991) -> (-10076.867872, -10022.531991)
  line L1239 (-10076.867872, -10022.531991) -> (-10076.867872, -10021.531991)
  line L1240 (-10075.437204, -10021.708318) -> (-10076.576815, -10021.708318)
  line L1241 (-10075.377984, -10021.531991) -> (-10075.437204, -10021.708318)
  line L1242 (-10076.867872, -10021.531991) -> (-10076.576815, -10021.708318)
  line L1243 (-10076.576815, -10021.708318) -> (-10076.576815, -10022.355664)
  line L1244 (-10076.867872, -10022.531991) -> (-10076.576815, -10022.355664)
  line L1245 (-10076.576815, -10022.355664) -> (-10075.437204, -10022.355664)
  line L1246 (-10075.377984, -10022.531991) -> (-10075.437204, -10022.355664)
  line L1247 (-10075.437204, -10022.355664) -> (-10075.437204, -10021.708318)
  ellipse E653 centre (-10076.296135, -10022.031991) end of major axis (-10076.296135, -10021.931991) minor radius 0.099326
  ellipse E654 centre (-10076.290339, -10022.031991) end of major axis (-10076.290339, -10021.931991) minor radius 0.099326 (-10076.290339, -10022.131991) -> (-10076.290339, -10021.931991) ccw
  line L1248 (-10076.290339, -10022.131991) -> (-10076.296135, -10022.131991)
  line L1249 (-10076.290339, -10021.931991) -> (-10076.296135, -10021.931991)
  line L1250 (-10076.129519, -10022.181991) -> (-10076.451159, -10022.181991)
  line L1251 (-10076.106335, -10022.181991) -> (-10076.129519, -10022.181991)
  line L1252 (-10076.451159, -10022.181991) -> (-10076.451159, -10021.881991)
  line L1253 (-10076.451159, -10021.881991) -> (-10076.129519, -10021.881991)
  line L1254 (-10076.106335, -10021.881991) -> (-10076.129519, -10021.881991)
  line L1255 (-10076.129519, -10021.881991) -> (-10076.129519, -10022.181991)
  line L1256 (-10076.106335, -10021.881991) -> (-10076.106335, -10022.181991)
  line L1257 (-10066.549515, -10020.046991) -> (-10066.549515, -10020.246991)
  line L1258 (-10066.711801, -10020.246991) -> (-10066.711801, -10020.046991)
  line L1259 (-10066.549515, -10020.246991) -> (-10066.711801, -10020.246991)
  line L1260 (-10066.463486, -10020.046991) -> (-10066.301201, -10020.046991)
  line L1261 (-10066.711801, -10020.046991) -> (-10066.463486, -10020.046991)
  line L1262 (-10067.70506, -10020.046991) -> (-10067.70506, -10020.246991)
  line L1263 (-10067.953374, -10020.046991) -> (-10067.70506, -10020.046991)
  line L1264 (-10066.549515, -10017.946991) -> (-10066.549515, -10018.146991)
  line L1265 (-10066.463486, -10018.146991) -> (-10066.711801, -10018.146991)
  line L1266 (-10066.711801, -10018.146991) -> (-10066.711801, -10017.946991)
  line L1267 (-10066.711801, -10017.946991) -> (-10066.549515, -10017.946991)
  line L1268 (-10066.301201, -10018.146991) -> (-10066.463486, -10018.146991)
  line L1269 (-10066.301201, -10018.146991) -> (-10066.301201, -10020.046991)
  line L1270 (-10066.711801, -10020.246991) -> (-10067.70506, -10020.246991)
  line L1271 (-10067.953374, -10020.046991) -> (-10067.953374, -10018.146991)
  line L1272 (-10066.463486, -10018.146991) -> (-10066.463486, -10020.046991)
  line L1273 (-10067.70506, -10017.946991) -> (-10066.711801, -10017.946991)
  line L1274 (-10067.70506, -10017.946991) -> (-10067.70506, -10018.146991)
  line L1275 (-10067.70506, -10018.146991) -> (-10067.953374, -10018.146991)
  line L1276 (-10067.70506, -10019.846991) -> (-10067.70506, -10018.346991)
  line L1277 (-10067.70506, -10018.346991) -> (-10066.711801, -10018.346991)
  line L1278 (-10066.711801, -10018.346991) -> (-10066.711801, -10019.846991)
  line L1279 (-10066.711801, -10019.846991) -> (-10067.70506, -10019.846991)
  line L1280 (-10067.414003, -10018.523318) -> (-10067.414003, -10019.670664)
  line L1281 (-10067.70506, -10018.346991) -> (-10067.414003, -10018.523318)
  line L1282 (-10067.70506, -10019.846991) -> (-10067.414003, -10019.670664)
  line L1283 (-10067.414003, -10019.670664) -> (-10066.771021, -10019.670664)
  line L1284 (-10066.711801, -10019.846991) -> (-10066.771021, -10019.670664)
  line L1285 (-10066.771021, -10019.670664) -> (-10066.771021, -10018.523318)
  line L1286 (-10066.711801, -10018.346991) -> (-10066.771021, -10018.523318)
  line L1287 (-10066.771021, -10018.523318) -> (-10067.414003, -10018.523318)
  ellipse E655 centre (-10067.121492, -10019.358902) end of major axis (-10067.121492, -10019.258902) minor radius 0.099326
  ellipse E656 centre (-10067.115696, -10019.358902) end of major axis (-10067.115696, -10019.258902) minor radius 0.099326 (-10067.115696, -10019.458902) -> (-10067.115696, -10019.258902) ccw
  line L1288 (-10067.115696, -10019.458902) -> (-10067.121492, -10019.458902)
  line L1289 (-10067.115696, -10019.258902) -> (-10067.121492, -10019.258902)
  line L1290 (-10066.966707, -10019.196991) -> (-10066.966707, -10019.520814)
  line L1291 (-10066.943523, -10019.520814) -> (-10066.966707, -10019.520814)
  line L1292 (-10066.943523, -10019.196991) -> (-10066.943523, -10019.520814)
  line L1293 (-10066.943523, -10019.196991) -> (-10066.966707, -10019.196991)
  line L1294 (-10066.966707, -10019.520814) -> (-10067.264685, -10019.520814)
  line L1295 (-10067.264685, -10019.520814) -> (-10067.264685, -10019.196991)
  line L1296 (-10067.264685, -10019.196991) -> (-10066.966707, -10019.196991)
  line L1297 (-10064.941411, -10013.746837) -> (-10064.918217, -10013.945353)
  line L1298 (-10064.918271, -10013.945494) -> (-10064.941481, -10013.746845)
  line L1299 (-10064.918217, -10013.945353) -> (-10064.918271, -10013.945494)
  line L1300 (-10064.69317, -10013.717834) -> (-10064.693115, -10013.717692)
  line L1301 (-10064.941481, -10013.746845) -> (-10064.69317, -10013.717834)
  line L1302 (-10065.934725, -10013.862893) -> (-10065.911515, -10014.061541)
  line L1303 (-10066.183036, -10013.891904) -> (-10065.934725, -10013.862893)
  line L1304 (-10066.383563, -10012.002274) -> (-10066.15523, -10011.975596)
  line L1305 (-10066.403525, -10012.004741) -> (-10066.403471, -10012.0046)
  line L1306 (-10066.178424, -10011.777081) -> (-10066.155214, -10011.97573)
  line L1307 (-10066.155214, -10011.97573) -> (-10066.403525, -10012.004741)
  line L1308 (-10066.178369, -10011.776939) -> (-10066.178424, -10011.777081)
  line L1309 (-10066.178369, -10011.776939) -> (-10065.185126, -10011.660892)
  line L1310 (-10064.913605, -10011.830529) -> (-10064.693115, -10013.717692)
  line L1311 (-10064.918271, -10013.945494) -> (-10065.911515, -10014.061541)
  line L1312 (-10066.183036, -10013.891904) -> (-10066.403525, -10012.004741)
  line L1313 (-10064.91366, -10011.830671) -> (-10064.69317, -10013.717834)
  line L1314 (-10066.178424, -10011.777081) -> (-10065.18518, -10011.661034)
  line L1315 (-10065.185126, -10011.660892) -> (-10065.161916, -10011.859541)
  line L1316 (-10065.161916, -10011.859541) -> (-10064.913605, -10011.830529)
  line L1317 (-10064.91366, -10011.830671) -> (-10065.161971, -10011.859682)
  line L1318 (-10065.161971, -10011.859682) -> (-10065.18518, -10011.661034)
  line L1319 (-10065.18518, -10011.661034) -> (-10065.185126, -10011.660892)
  line L1320 (-10065.161971, -10011.859682) -> (-10065.161916, -10011.859541)
  line L1321 (-10064.913605, -10011.830529) -> (-10064.91366, -10011.830671)
  line L1322 (-10065.957934, -10013.664244) -> (-10066.132005, -10012.174378)
  line L1323 (-10066.132005, -10012.174378) -> (-10065.138761, -10012.058331)
  line L1324 (-10065.138761, -10012.058331) -> (-10064.96469, -10013.548197)
  line L1325 (-10064.96469, -10013.548197) -> (-10065.957934, -10013.664244)
  line L1326 (-10065.936368, -10012.328951) -> (-10065.803222, -10013.468545)
  line L1327 (-10066.132005, -10012.174378) -> (-10065.936368, -10012.328951)
  line L1328 (-10065.957934, -10013.664244) -> (-10065.803222, -10013.468545)
  line L1329 (-10065.803222, -10013.468545) -> (-10065.160249, -10013.393422)
  line L1330 (-10064.96469, -10013.548197) -> (-10065.160249, -10013.393422)
  line L1331 (-10065.160249, -10013.393422) -> (-10065.293396, -10012.253828)
  line L1332 (-10065.138761, -10012.058331) -> (-10065.293396, -10012.253828)
  line L1333 (-10065.293396, -10012.253828) -> (-10065.936368, -10012.328951)
  circle A27 centre (-10065.517924, -10013.121353) radius 0.1
  line L1334 (-10065.387725, -10012.943124) -> (-10065.350146, -10013.264759)
  line L1335 (-10065.350139, -10013.264739) -> (-10065.350146, -10013.264759)
  line L1336 (-10065.387717, -10012.943104) -> (-10065.350139, -10013.264739)
  line L1337 (-10065.387717, -10012.943104) -> (-10065.387725, -10012.943124)
  line L1338 (-10065.350146, -10013.264759) -> (-10065.64812, -10013.299573)
  line L1339 (-10065.64812, -10013.299573) -> (-10065.685698, -10012.977938)
  line L1340 (-10065.685691, -10012.977918) -> (-10065.685698, -10012.977938)
  line L1341 (-10065.685698, -10012.977938) -> (-10065.387725, -10012.943124)
  line L1342 (-10065.685691, -10012.977918) -> (-10065.387717, -10012.943104)
  line L1343 (-10079.603594, -10026.293678) -> (-10079.802686, -10026.274807)
  line L1344 (-10079.802692, -10026.274707) -> (-10079.603585, -10026.293579)
  line L1345 (-10079.802686, -10026.274807) -> (-10079.802692, -10026.274707)
  line L1346 (-10079.627175, -10026.542464) -> (-10079.627169, -10026.542564)
  line L1347 (-10079.603585, -10026.293579) -> (-10079.627175, -10026.542464)
  line L1348 (-10079.509221, -10025.298042) -> (-10079.708329, -10025.279169)
  line L1349 (-10079.485631, -10025.049157) -> (-10079.509221, -10025.298042)
  line L1350 (-10079.407047, -10026.563429) -> (-10079.627169, -10026.542564)
  line L1351 (-10079.802692, -10026.274707) -> (-10079.708329, -10025.279169)
  line L1352 (-10079.485631, -10025.049157) -> (-10077.594109, -10025.228447)
  line L1353 (-10077.874828, -10026.708562) -> (-10079.627175, -10026.542464)
  line L1354 (-10077.418592, -10025.496204) -> (-10077.433041, -10025.648641)
  line L1355 (-10077.594109, -10025.228447) -> (-10077.594103, -10025.228547)
  line L1356 (-10077.418592, -10025.496204) -> (-10077.6177, -10025.477332)
  line L1357 (-10077.6177, -10025.477332) -> (-10077.594109, -10025.228447)
  line L1358 (-10077.418586, -10025.496304) -> (-10077.418592, -10025.496204)
  line L1359 (-10079.310114, -10025.316914) -> (-10077.816807, -10025.458459)
  line L1360 (-10077.816807, -10025.458459) -> (-10077.91117, -10026.453997)
  line L1361 (-10077.91117, -10026.453997) -> (-10079.404477, -10026.312452)
  line L1362 (-10079.404477, -10026.312452) -> (-10079.310114, -10025.316914)
  line L1363 (-10078.008982, -10025.617432) -> (-10079.151208, -10025.509165)
  line L1364 (-10077.816807, -10025.458459) -> (-10078.008982, -10025.617432)
  line L1365 (-10079.310114, -10025.316914) -> (-10079.151208, -10025.509165)
  line L1366 (-10079.151208, -10025.509165) -> (-10079.212294, -10026.153622)
  line L1367 (-10079.404477, -10026.312452) -> (-10079.212294, -10026.153622)
  line L1368 (-10079.212294, -10026.153622) -> (-10078.070067, -10026.261889)
  line L1369 (-10077.91117, -10026.453997) -> (-10078.070067, -10026.261889)
  line L1370 (-10078.070067, -10026.261889) -> (-10078.008982, -10025.617432)
  circle A28 centre (-10078.871381, -10025.860794) radius 0.1
  line L1371 (-10078.724347, -10026.025407) -> (-10079.046725, -10025.99485)
  line L1372 (-10078.724346, -10026.025422) -> (-10079.046724, -10025.994865)
  line L1373 (-10079.046725, -10025.99485) -> (-10079.018416, -10025.696189)
  line L1374 (-10079.018416, -10025.696189) -> (-10078.696038, -10025.726746)
  line L1375 (-10078.696038, -10025.726746) -> (-10078.724347, -10026.025407)
  line L1376 (-10068.99061, -10024.803404) -> (-10068.990604, -10024.803504)
  line L1377 (-10069.009483, -10025.002511) -> (-10068.99061, -10024.803404)
  line L1378 (-10069.009477, -10025.002612) -> (-10069.009483, -10025.002511)
  line L1379 (-10068.741726, -10024.826995) -> (-10068.74172, -10024.827095)
  line L1380 (-10068.99061, -10024.803404) -> (-10068.741726, -10024.826995)
  line L1381 (-10070.005021, -10024.908148) -> (-10070.005014, -10024.908249)